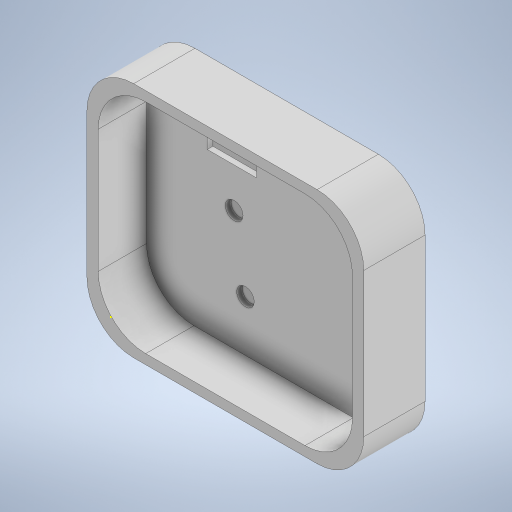
# Autodesk Inventor part: Bottom_Housing_K30
Saved by Autodesk Inventor 2023 (Build 270158000, 158)
## iProperties
Created: 2022-06-02
Part Number: Bottom_Housing_K30
Material: Generic
Document SubType Name: Modeling
Designer: djp6984
Density: 1 g/cm^3
Appearance: Default
Author: djp6984
Autodesk Inventor part; units mm, degrees
ref_plane "YZ Plane" through (0, 0, 0) normal (1, 0, 0) x (0, 1, 0)
ref_plane "XZ Plane" through (0, 0, 0) normal (0, 1, 0) x (-1, 0, 0)
ref_plane "XY Plane" through (0, 0, 0) normal (0, 0, 1) x (1, 0, 0)
sketch "Sketch1" plane through (0, 0, 0) normal (0, 0, 1) x (1, 0, 0)
  line L0 (0, 0) -> (72.136, 0)
  line L1 (72.136, 0) -> (72.136, 59.69)
  line L2 (72.136, 59.69) -> (0, 59.69)
  line L3 (0, 59.69) -> (0, 0)
  dimension "d0" = 59.69
  dimension "d1" = 72.136
  constraints: 8 end point, 2 parallel, 1 horizontal, 1 perpendicular
  measures "d0" distance of L0.end L1.end
  measures "d1" distance of L1.end L2.end
extrude "Extrusion1" add sketch "Sketch1" along normal blind 21.844
sketch "Sketch2" plane through (0, 0, 21.844) normal (0, 0, 1) x (1, 0, 0)
  line L0 (3.048, 56.642) -> (69.088, 56.642)
  line L1 (69.088, 56.642) -> (69.088, 3.048)
  line L2 (69.088, 3.048) -> (3.048, 3.048)
  line L3 (3.048, 3.048) -> (3.048, 56.642)
  line L4 (72.136, 59.69) -> (0, 59.69) projected
  line L5 (72.136, 0) -> (72.136, 59.69) projected
  line L6 (0, 0) -> (72.136, 0) projected
  line L7 (0, 59.69) -> (0, 0) projected
  dimension "d4" = 3.048
  dimension "d5" = 3.048
  dimension "d6" = 3.048
  dimension "d7" = 3.048
  constraints: 8 end point, 2 parallel, 1 horizontal, 1 perpendicular
  measures "d4" distance between parallel lines of L4 L0
  measures "d5" distance between parallel lines of L5 L1
  measures "d6" distance between parallel lines of L6 L2
  measures "d7" distance between parallel lines of L7 L3
extrude "Extrusion2" cut sketch "Sketch2" against normal blind 15.24 contours L0 L1 L2 L3
sketch "Sketch3" plane through (0, 0, 6.604) normal (0, 0, 1) x (1, 0, 0)
  line L0 (15.113, 45.72) -> (30.607, 45.72)
  line L1 (30.607, 45.72) -> (30.607, 51.689)
  line L2 (30.607, 51.689) -> (15.113, 51.689)
  line L3 (15.113, 51.689) -> (15.113, 45.72)
  line L4 (3.048, 56.642) -> (69.088, 56.642) projected
  line L5 (3.048, 3.048) -> (3.048, 56.642) projected
  circle A0 centre (23.622, 33.274) radius 2.794
  circle A1 centre (27.178, 11.5062) radius 2.794
  point P0 (0, 0)
  dimension "d10" = 5.969
  dimension "d11" = 15.494
  dimension "d12" = 4.953
  dimension "d13" = 12.065
  dimension "d14" = 5.588
  dimension "d15" = 5.588
  dimension "d17" = 24.13
  dimension "d18" = 20.574
  dimension "d21" = 23.368
  dimension "d22" = 45.1358
  constraints: 8 end point, 2 centre point, 2 parallel, 1 horizontal, 1 perpendicular
  measures "d10" distance of L0.end L1.end
  measures "d11" distance of L0.start L0.end
  measures "d12" distance between parallel lines of L4 L2
  measures "d13" distance between parallel lines of L5 L3
  measures "d14" diameter of A1
  measures "d15" diameter of A0
  measures "d17" distance from line of L5 A1.centre
  measures "d18" distance from line of L5 A0.centre
  measures "d21" distance from line of L4 A0.centre
  measures "d22" distance from line of L4 A1.centre
extrude "Extrusion3" cut sketch "Sketch3" against normal blind 1.778
sketch "Sketch4" plane through (0, 0, 21.844) normal (0, 0, 1) x (1, 0, 0)
  point P0 (0, 0)
sketch "Sketch5" plane through (0, 0, 21.844) normal (0, 0, 1) x (1, 0, 0)
  line L0 (-2.54, -2.54) -> (74.676, -2.54)
  line L1 (74.676, -2.54) -> (74.676, 62.23)
  line L2 (74.676, 62.23) -> (-2.54, 62.23)
  line L3 (-2.54, 62.23) -> (-2.54, -2.54)
  line L4 (72.136, 0) -> (72.136, 59.69) projected
  line L5 (72.136, 59.69) -> (0, 59.69) projected
  line L6 (0, 59.69) -> (0, 0) projected
  line L7 (0, 0) -> (72.136, 0) projected
  line L8 (0, 0) -> (72.136, 0)
  line L9 (72.136, 0) -> (72.136, 59.69)
  line L10 (72.136, 59.69) -> (0, 59.69)
  line L11 (0, 59.69) -> (0, 0)
  dimension "d23" = 2.54
  dimension "d24" = 2.54
  dimension "d25" = 2.54
  dimension "d26" = 2.54
  constraints: 16 end point, 4 parallel, 2 horizontal, 2 perpendicular
  measures "d23" distance between parallel lines of L1 L4
  measures "d24" distance between parallel lines of L2 L5
  measures "d25" distance between parallel lines of L6 L3
  measures "d26" distance between parallel lines of L0 L7
extrude "Extrusion4" add sketch "Sketch5" against normal blind 21.844
sketch "Sketch6" plane through (0, 0, 21.844) normal (0, 0, 1) x (1, 0, 0)
  line L0 (-0.762, -0.762) -> (72.898, -0.762)
  line L1 (72.898, -0.762) -> (72.898, 60.452)
  line L2 (72.898, 60.452) -> (-0.762, 60.452)
  line L3 (-0.762, 60.452) -> (-0.762, -0.762)
  line L4 (3.048, 3.048) -> (3.048, 56.642) projected
  line L5 (3.048, 56.642) -> (69.088, 56.642) projected
  line L6 (69.088, 56.642) -> (69.088, 3.048) projected
  line L7 (69.088, 3.048) -> (3.048, 3.048) projected
  point P0 (0, 0)
  dimension "d29" = 3.81
  dimension "d30" = 3.81
  dimension "d31" = 3.81
  dimension "d32" = 3.81
  constraints: 8 end point, 2 parallel, 1 horizontal, 1 perpendicular
  measures "d29" distance between parallel lines of L4 L3
  measures "d30" distance between parallel lines of L5 L2
  measures "d31" distance between parallel lines of L6 L1
  measures "d32" distance between parallel lines of L7 L0
extrude "Extrusion5" cut sketch "Sketch6" against normal blind 15.24
sketch "Sketch7" plane through (0, 0, 21.844) normal (0, 0, 1) x (1, 0, 0)
  point P0 (0, 0)
sketch "Sketch8" plane through (0, 0, 21.844) normal (0, 0, 1) x (1, 0, 0)
  line L0 (74.676, -2.54) -> (-2.54, -2.54) projected
  line L1 (-2.54, -2.54) -> (74.676, -2.54)
  line L2 (74.676, -2.54) -> (74.676, 62.23)
  line L3 (74.676, 62.23) -> (-2.54, 62.23)
  line L4 (-2.54, 62.23) -> (-2.54, -2.54)
  line L5 (-7.62, -7.62) -> (79.756, -7.62)
  line L6 (79.756, -7.62) -> (79.756, 67.31)
  line L7 (79.756, 67.31) -> (-7.62, 67.31)
  line L8 (-7.62, 67.31) -> (-7.62, -7.62)
  point P0 (0, 0)
  dimension "d35" = 5.08
  dimension "d36" = 5.08
  dimension "d37" = 5.08
  dimension "d38" = 5.08
  constraints: 16 end point, 4 parallel, 2 horizontal, 2 perpendicular
  measures "d35" distance between parallel lines of L4 L8
  measures "d36" distance between parallel lines of L7 L3
  measures "d37" distance between parallel lines of L6 L2
  measures "d38" distance between parallel lines of L5 L0
extrude "Extrusion6" add sketch "Sketch8" against normal blind 21.844
sketch "Sketch10" plane through (0, 0, 21.844) normal (0, 0, 1) x (1, 0, 0)
  point P0 (0, 0)
sketch "Sketch15" plane through (0, 0, 21.844) normal (0, 0, 1) x (1, 0, 0)
  line L0 (72.898, -0.762) -> (-0.762, -0.762) projected
  line L1 (-0.762, 60.452) -> (72.898, 60.452) projected
  line L2 (-0.762, -0.762) -> (72.898, -0.762)
  line L3 (72.898, -0.762) -> (72.898, 60.452)
  line L4 (72.898, 60.452) -> (-0.762, 60.452)
  line L5 (-0.762, 60.452) -> (-0.762, -0.762)
  line L6 (70.358, 57.912) -> (1.778, 57.912)
  line L7 (1.778, 57.912) -> (1.778, 1.778)
  line L8 (1.778, 1.778) -> (70.358, 1.778)
  line L9 (70.358, 1.778) -> (70.358, 57.912)
  point P0 (0, 0)
  dimension "d63" = 2.54
  dimension "d64" = 2.54
  dimension "d65" = 2.54
  dimension "d66" = 2.54
  constraints: 16 end point, 4 parallel, 2 horizontal, 2 perpendicular
  measures "d63" distance between parallel lines of L1 L6
  measures "d64" distance between parallel lines of L7 L5
  measures "d65" distance between parallel lines of L0 L8
  measures "d66" distance between parallel lines of L3 L9
extrude "Extrusion8" add sketch "Sketch15" against normal blind 15.24
sketch "Sketch16" plane through (0, 0, 21.844) normal (0, 0, 1) x (1, 0, 0)
  line L0 (10.922, -4.572) -> (61.214, -4.572)
  line L1 (76.2, 10.414) -> (76.2, 49.276)
  line L2 (61.214, 64.262) -> (10.922, 64.262)
  line L3 (-4.064, 49.276) -> (-4.064, 10.414)
  line L4 (1.778, 57.912) -> (70.358, 57.912) projected
  line L5 (70.358, 1.778) -> (1.778, 1.778) projected
  line L6 (1.778, 1.778) -> (1.778, 57.912) projected
  line L7 (70.358, 57.912) -> (70.358, 1.778) projected
  line L8 (1.778, 57.912) -> (1.778, 1.778) projected
  line L9 (70.358, 1.778) -> (70.358, 57.912) projected
  line L10 (1.778, 1.778) -> (70.358, 1.778)
  line L11 (70.358, 1.778) -> (70.358, 57.912)
  line L12 (70.358, 57.912) -> (1.778, 57.912)
  line L13 (1.778, 57.912) -> (1.778, 1.778)
  arc A0 (-4.064, 10.414) -> (10.922, -4.572) centre (10.922, 10.414) ccw
  arc A1 (10.922, 64.262) -> (-4.064, 49.276) centre (10.922, 49.276) ccw
  arc A2 (76.2, 49.276) -> (61.214, 64.262) centre (61.214, 49.276) ccw
  arc A3 (61.214, -4.572) -> (76.2, 10.414) centre (61.214, 10.414) ccw
  point P0 (0, 0)
  dimension "d69" = 6.35
  dimension "d70" = 6.35
  dimension "d71" = 5.842
  dimension "d72" = 5.842
  dimension "d73" = 14.986
  constraints: 16 end point, 8 point on circle, 8 tangent, 4 centre point, 4 parallel, 3 equal radius, 2 horizontal, 2 perpendicular
  measures "d69" distance between parallel lines of L4 L2
  measures "d70" distance between parallel lines of L5 L0
  measures "d71" distance between parallel lines of L6 L3
  measures "d72" distance between parallel lines of L7 L1
  measures "d73" radius of A0
extrude "Extrusion9" cut sketch "Sketch16" against normal blind 15.24
fillet "Fillet2" radius 14.732 4 edges at (79.756, 67.31, 10.922) (79.756, -7.62, 10.922) (-7.62, 67.31, 10.922) (-7.62, -7.62, 10.922)
sketch "Sketch17" plane through (0, 0, 0) normal (0, 0, -1) x (-1, 0, 0)
  line L0 (-94.7004, 78.8948) -> (24.3491, 78.8948)
  line L1 (24.3491, 78.8948) -> (24.3491, -15.2836)
  line L2 (24.3491, -15.2836) -> (-94.7004, -15.2836)
  line L3 (-94.7004, -15.2836) -> (-94.7004, 78.8948)
  point P0 (0, 0)
  constraints: 8 end point, 2 parallel, 1 horizontal, 1 perpendicular
extrude "Extrusion10" cut sketch "Sketch17" against normal blind 2.5
body "Solid1"
